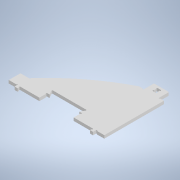
# Autodesk Inventor part: Support E
Saved by Autodesk Inventor 2020 (Build 240168000, 168)
## iProperties
Created: 2020-03-07
Part Number: Support E
Material: Generic
Document SubType Name: Modeling
Designer: Daniel Wikman
Density: 1 g/cm^3
Appearance: Default
Author: Daniel Wikman
Autodesk Inventor part; units mm, degrees
ref_plane "YZ Plane" through (0, 0, 0) normal (1, 0, 0) x (0, 1, 0)
ref_plane "XZ Plane" through (0, 0, 0) normal (0, 1, 0) x (-1, 0, 0)
ref_plane "XY Plane" through (0, 0, 0) normal (0, 0, 1) x (1, 0, 0)
sketch "Sketch1" plane through (0, 0, 0) normal (0, 1, 0) x (-1, 0, 0)
  line L0 (113.8016, -163.8079) -> (118.6285, -172.1682)
  line L1 (113.8016, -163.8079) -> (118.4883, -163.8079)
  line L2 (118.4883, -148.1364) -> (118.4883, -161.1412)
  line L3 (156.6836, -142.6364) -> (162.6836, -142.6364)
  line L4 (162.6836, -142.6364) -> (162.6836, -148.1364)
  line L5 (156.6866, -148.1364) -> (118.4883, -148.1364)
  line L6 (11.6836, -145.4697) -> (11.6846, -142.6364)
  line L7 (11.6846, -142.6364) -> (5.6846, -142.6364)
  line L8 (5.6846, -142.6364) -> (5.6845, -148.1281)
  line L9 (11.6831, -148.1364) -> (49.8814, -148.1364)
  arc A0 (11.6836, -145.4697) -> (11.6831, -148.1364) centre (11.6831, -146.803) ccw
  arc A1 (3.0194, -148.0629) -> (5.6845, -148.1281) centre (4.3512, -148.1281) ccw
  line L10 (-11.4601, -148.0629) -> (3.0194, -148.0629)
  line L11 (162.6836, -145.3864) -> (185.043, -145.3864) construction
  line L12 (156.6836, -142.6364) -> (156.6836, -145.4697)
  line L13 (165.3503, -148.1364) -> (179.8299, -148.1364)
  arc A2 (156.6866, -148.1364) -> (156.6836, -145.4697) centre (156.6836, -146.803) ccw
  arc A3 (162.6836, -148.1364) -> (165.3503, -148.1364) centre (164.017, -148.1364) ccw
  line L14 (179.8299, -148.1364) -> (179.8299, -171.4697)
  line L15 (179.8299, -171.4697) -> (162.6836, -171.4697)
  line L16 (118.4883, -161.1412) -> (118.4883, -164.2811)
  arc A4 (118.4883, -163.8079) -> (118.4883, -161.1412) centre (118.4883, -162.4745) ccw
  line L17 (84.1849, -148.1364) -> (84.1849, -155.2534)
  arc A5 (117.4738, -174.1682) -> (118.6285, -172.1682) centre (117.4738, -172.8349) ccw
  line L18 (84.1849, -174.1682) -> (117.4738, -174.1682)
  line L19 (54.5681, -163.8079) -> (49.7413, -172.1682)
  line L20 (54.5681, -163.8079) -> (49.8814, -163.8079)
  line L21 (49.8814, -148.1364) -> (49.8814, -161.1412)
  line L22 (49.8814, -161.1412) -> (49.8814, -164.2811)
  arc A6 (49.8814, -161.1412) -> (49.8814, -163.8079) centre (49.8814, -162.4745) ccw
  arc A7 (49.7413, -172.1682) -> (50.896, -174.1682) centre (50.896, -172.8349) ccw
  line L23 (84.1849, -174.1682) -> (50.896, -174.1682)
  line L24 (-11.4601, -148.0629) -> (-11.4601, -267.5629)
  line L25 (-11.4601, -267.5629) -> (-4.1268, -267.5629)
  arc A8 (-1.4601, -267.5629) -> (-4.1268, -267.5629) centre (-2.7935, -267.5629) ccw
  line L26 (-1.4601, -267.5629) -> (-1.4601, -286.2296)
  line L27 (-0.1268, -287.5629) -> (13.5398, -287.5629)
  arc A9 (-1.4601, -286.2296) -> (-0.1268, -287.5629) centre (-0.1268, -286.2296) ccw
  line L28 (38.5397, -267.5629) -> (31.2064, -267.5629)
  arc A10 (31.2064, -267.5629) -> (28.5397, -267.5629) centre (29.873, -267.5629) ccw
  line L29 (28.5397, -267.5629) -> (28.5397, -286.2296)
  line L30 (27.2064, -287.5629) -> (13.5398, -287.5629)
  arc A11 (27.2064, -287.5629) -> (28.5397, -286.2296) centre (27.2064, -286.2296) ccw
  line L31 (13.5398, -267.5629) -> (13.5398, -273.0629) construction
  line L32 (16.7898, -273.0629) -> (10.2898, -273.0629)
  line L33 (10.2898, -275.7296) -> (10.2898, -280.3963)
  line L34 (10.2898, -283.0629) -> (16.7898, -283.0629)
  line L35 (16.7898, -280.3963) -> (16.7898, -275.7296)
  arc A12 (16.7898, -275.7296) -> (16.7898, -273.0629) centre (16.7898, -274.3963) ccw
  arc A13 (10.2898, -273.0629) -> (10.2898, -275.7296) centre (10.2898, -274.3963) ccw
  arc A14 (10.2898, -280.3963) -> (10.2898, -283.0629) centre (10.2898, -281.7296) ccw
  arc A15 (16.7898, -283.0629) -> (16.7898, -280.3963) centre (16.7898, -281.7296) ccw
  arc A16 (38.5397, -267.5629) -> (162.6836, -171.4697) centre (-155.0558, 110.7832) ccw
  point P0 (-1.4601, -287.5629)
  dimension "d170" = 13.0048
  dimension "d173" = 6
  dimension "d174" = 5.5
  dimension "d202" = 6
  dimension "d203" = 1.3333
  dimension "d204" = 1.3333
  dimension "d208" = 191.29
  dimension "d209" = 2.6667
  dimension "d210" = 2.6667
  dimension "d212" = 14.4796
  dimension "d213" = 61.3416
  dimension "d214" = 145
  dimension "d223" = 38.1984
  dimension "d226" = 61.3416
  dimension "d232" = 2.6667
  dimension "d233" = 2.6667
  dimension "d235" = 60
  dimension "d236" = 33.2889
  dimension "d238" = 68.6068
  dimension "d239" = 33.2889
  dimension "d242" = 119.5
  dimension "d243" = 7.3333
  dimension "d244" = 2.6667
  dimension "d245" = 20
  dimension "d246" = 1.3333
  dimension "d247" = 5.5
  dimension "d248" = 4.5
  dimension "d249" = 6.5
  dimension "d250" = 3.25
  dimension "d251" = 10
  dimension "d252" = 2.6667
  dimension "d253" = 2.6667
  dimension "d254" = 2.6667
  dimension "d255" = 2.6667
  dimension "d256" = 425
  constraints: 73 end point, 35 point on circle, 17 centre point, 16 point on line, 4 horizontal, 4 vertical, 2 parallel, 2 tangent, 1 midpoint, 1 perpendicular, 3 other
  measures "d170" distance of L2.start L2.end
  measures "d173" distance of L3.start L3.end
  measures "d174" distance of L4.end L3.end
  measures "d202" distance of L6.end L7.end
  measures "d203" radius of A0
  measures "d204" radius of A1
  measures "d208" distance of L10.start L13.end
  measures "d209" diameter of A2
  measures "d210" diameter of A3
  measures "d212" distance of L10.start L10.end
  measures "d213" distance from line of L13.end L2
  measures "d214" distance from line of L6.start L12
  measures "d223" distance of L9.start L9.end
  measures "d226" distance of L9.end L10.start
  measures "d232" diameter of A4
  measures "d233" diameter of A5
  measures "d235" angle of L18 L0
  measures "d236" distance of L18.start L18.end
  measures "d238" diameter of L21 L17
  measures "d239" distance of L18.start L23.end
  measures "d242" distance of L10.start L24.end
  measures "d243" distance of L24.end L25.end
  measures "d244" diameter of A8
  measures "d245" distance of L26.start point (-1.46, -287.563)
  measures "d246" radius of A9
  measures "d247" distance of L31.start L31.end
  measures "d248" distance between parallel lines of L27 L34
  measures "d249" distance of L32.start L32.end
  measures "d250" distance between parallel lines of L31 L35
  measures "d251" distance of L34.end L32.start
  measures "d252" diameter of A12
  measures "d253" diameter of A13
  measures "d254" diameter of A14
  measures "d255" diameter of A15
  measures "d256" radius of A16
extrude "Extrusion5" add sketch "Sketch1" along normal blind 6 contours L1 A4 L2 L5 A2 L12 L3 L4 A3 L13 L14 L15 A16 L28 A10 L29 A11 L30 L27 A9 L26 A8 L25 L24 L10 A1 L8 L7 L6 A0 L9 L21 A6 L20 L19 A7 L23 L18 A5 L0
body "Solid5"
